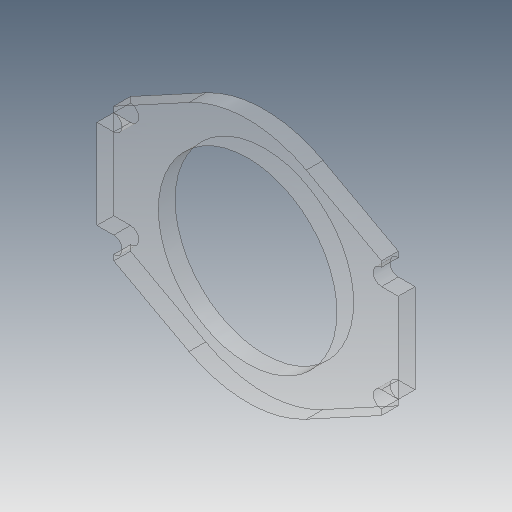
# Autodesk Inventor part: RS555-71K_MotorsupportPolica
Saved by Autodesk Inventor 2019.4 (Build 234330000, 330)
## iProperties
Created: 2019-06-14
Part Number: RS555-71K_MotorsupportPolica
Material: ポリカーボネート、クリア
Document SubType Name: Modeling
Designer: AzLIer
Density: 1.2 g/cm^3
Appearance: ポリカーボネート - クリア
Mass: 3.64035 g
Surface Area: 28.4026 cm^2
Volume: 3.03362 cm^3
Author: AzLIer
Autodesk Inventor part; units mm, degrees
ref_plane "YZ Plane" through (0, 0, 0) normal (1, 0, 0) x (0, 1, 0)
ref_plane "XZ Plane" through (0, 0, 0) normal (0, 1, 0) x (-1, 0, 0)
ref_plane "XY Plane" through (0, 0, 0) normal (0, 0, 1) x (1, 0, 0)
sketch "スケッチ1" plane through (0, 0, 0) normal (0, 0, 1) x (1, 0, 0)
  circle A0 centre (0, 0) radius 16
  circle A1 centre (0, 0) radius 22
  dimension "d0" = 32
  dimension "d7" = 6
  constraints: 2 centre point, 1 coincident
  measures "d0" diameter of A0
  measures "d7" radial gap between concentric circles of A0 A1
extrude "押し出し1" add sketch "スケッチ1" along normal blind 3
sketch "スケッチ2" plane through (0, 0, 0) normal (0, 0, -1) x (-1, 0, 0)
  line L0 (-27, 8) -> (-27, -8)
  line L1 (27, -8) -> (27, 8)
  line L2 (24, -8) -> (27, -8)
  line L3 (-27, -8) -> (-24, -8)
  line L4 (-24, 8) -> (-27, 8)
  line L5 (27, 8) -> (24, 8)
  line L6 (-24, 12) -> (-24, 11)
  line L7 (-24, -11) -> (-24, -12)
  line L8 (24, -12) -> (24, -11)
  line L9 (24, 11) -> (24, 12)
  line L10 (-24, -12) -> (-10.5005, -19.3323)
  line L11 (10.5005, -19.3323) -> (24, -12)
  line L12 (24, 12) -> (10.5005, 19.3323)
  line L13 (-10.5005, 19.3323) -> (-24, 12)
  circle A0 centre (0, 0) radius 22 projected
  arc A1 (24, -8) -> (24, -11) centre (24, -9.5) ccw
  arc A2 (24, 11) -> (24, 8) centre (24, 9.5) ccw
  arc A3 (-24, 8) -> (-24, 11) centre (-24, 9.5) ccw
  arc A4 (-24, -11) -> (-24, -8) centre (-24, -9.5) ccw
  point P0 (-27, 0)
  point P1 (27, 0)
  dimension "d10" = 54
  dimension "d11" = 16
  dimension "d13" = 48
  dimension "d14" = 24
  dimension "d17" = 3
  constraints: 28 end point, 12 point on circle, 10 parallel, 8 point on line, 5 equal length, 5 tangent, 4 centre point, 3 equal radius, 3 horizontal alignment, 2 horizontal, 2 midpoint, 2 perpendicular, 1 vertical
  measures "d10" distance of L1.start L0.end
  measures "d11" distance of L0.end L0.start
  measures "d13" distance of L7.end L8.start
  measures "d14" distance of L6.start L7.end
  measures "d17" diameter of A4
extrude "押し出し2" add sketch "スケッチ2" against normal blind 3 contours L4 A3 L6 L13 A0 L10 L7 A4 L3 L0 | L12 L9 A2 L5 L1 L2 A1 L8 L11 A0
